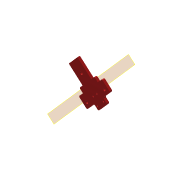
# Autodesk Inventor part: Neje_Base_Slide_y
Saved by Autodesk Inventor 2019.4 (Build 234330000, 330)
## iProperties
Created: 2021-04-08
Part Number: Neje_Base_Slide_y
Material: Generic
Document SubType Name: Modeling
Designer: diederichbenedict
Density: 1 g/cm^3
Appearance: Light Red
Author: diederichbenedict
Autodesk Inventor part; units mm, degrees
ref_plane "YZ Plane" through (0, 0, 0) normal (1, 0, 0) x (0, 1, 0)
ref_plane "XZ Plane" through (0, 0, 0) normal (0, 1, 0) x (-1, 0, 0)
ref_plane "XY Plane" through (0, 0, 0) normal (0, 0, 1) x (1, 0, 0)
ref_plane "Work Plane1" through (-54.8706, 13.9436, 0) normal (0, 0, 1) x (0.7510442, -0.660252, 0)
sketch "Sketch1" plane through (-54.8706, 13.9436, 0) normal (0, 0, 1) x (0.7510442, -0.660252, 0)
  line L0 (-38.2203, 53.235) -> (-38.2203, 65.735)
  line L1 (-38.2203, 65.735) -> (-3.2203, 65.735)
  line L2 (-3.2203, 65.735) -> (-3.2203, 72.735)
  line L3 (-1.2203, 74.735) -> (5.4797, 74.735)
  line L4 (5.4797, 74.735) -> (5.4797, 84.735)
  line L5 (7.4797, 86.735) -> (24.3797, 86.735)
  line L6 (26.3797, 84.735) -> (26.3797, 67.935)
  line L7 (28.3797, 65.935) -> (35.0797, 65.935)
  line L8 (37.0797, 63.935) -> (37.0797, 53.235)
  arc A0 (37.0797, 63.935) -> (35.0797, 65.935) centre (35.0797, 63.935) ccw
  arc A1 (26.3797, 67.935) -> (28.3797, 65.935) centre (28.3797, 67.935) ccw
  arc A2 (26.3797, 84.735) -> (24.3797, 86.735) centre (24.3797, 84.735) ccw
  arc A3 (7.4797, 86.735) -> (5.4797, 84.735) centre (7.4797, 84.735) ccw
  arc A4 (-1.2203, 74.735) -> (-3.2203, 72.735) centre (-1.2203, 72.735) ccw
  circle A5 centre (30.6297, 61.785) radius 1.6
  circle A6 centre (16.7597, 58.485) radius 1.6
  circle A7 centre (18.5797, 78.435) radius 2.5
  circle A8 centre (-17.6203, 53.235) radius 2.5
  line L9 (37.0797, 53.235) -> (-15.1203, 53.235)
  line L10 (-20.1203, 53.235) -> (-38.2203, 53.235)
  point P0 (50.4165, 25.7562)
  dimension "d1" = 35
  dimension "d2" = 9
  dimension "d3" = 8.7
  dimension "d4" = 12
  dimension "d5" = 20.9
  dimension "d6" = 20.8
  dimension "d7" = 10.7
  dimension "d8" = 2
  dimension "d9" = 3.2
  dimension "d10" = 3.2
  dimension "d11" = 5
  dimension "d12" = 5
  dimension "d13" = 20.6
  dimension "d14" = 7.8
  dimension "d15" = 8.3
  dimension "d16" = 4.15
  dimension "d17" = 6.45
  dimension "d18" = 20.32
  constraints: 22 end point, 12 point on circle, 11 perpendicular, 10 tangent, 9 centre point, 4 equal radius, 2 horizontal
  measures "d1" distance between parallel lines of L2 L0
  measures "d2" distance between parallel lines of L1 L3
  measures "d3" distance between parallel lines of L4 L2
  measures "d4" distance between parallel lines of L3 L5
  measures "d5" distance between parallel lines of L6 L4
  measures "d6" distance between parallel lines of L7 L5
  measures "d7" distance between parallel lines of L8 L6
  measures "d8" radius of A0
  measures "d9" diameter of A5
  measures "d10" diameter of A6
  measures "d11" diameter of A7
  measures "d12" diameter of A8
  measures "d13" distance from line of A8.centre L0
  measures "d14" distance from line of A7.centre L6
  measures "d15" distance from line of A7.centre L5
  measures "d16" distance from line of A5.centre L7
  measures "d17" distance from line of A5.centre L8
  measures "d18" distance from line of A6.centre L8
extrude "Extrusion1" add sketch "Sketch1" along normal blind 4.7 contours L0 L1 L2 A4 L3 L4 A3 L5 A2 L6 A1 L7 A0 L8 L9 A8 L10
mirror "Mirror1" about plane through (-31.078, 63.9086, 0) normal (-0.660252, -0.7510442, 0) of "Extrusion1"
body "Solid1"
